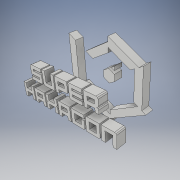
# Autodesk Inventor part: Super-Haxagon
Saved by Autodesk Inventor 2017 (Build 210142000, 142)
## iProperties
Created: 2016-12-10
Part Number: Super-Haxagon
Material: Generic
Document SubType Name: Modeling
Designer: AJ
Density: 1 g/cm^3
Appearance: Default
Author: AJ
Autodesk Inventor part; units mm, degrees
ref_plane "YZ Plane" through (0, 0, 0) normal (1, 0, 0) x (0, 1, 0)
ref_plane "XZ Plane" through (0, 0, 0) normal (0, 1, 0) x (-1, 0, 0)
ref_plane "XY Plane" through (0, 0, 0) normal (0, 0, 1) x (1, 0, 0)
sketch "Shapes" plane through (0, 0, 0) normal (0, 0, 1) x (1, 0, 0)
  circle A0 centre (0, 0) radius 19.05 construction
  line L0 (15.6048, 10.9266) -> (-1.6603, 18.9775)
  line L1 (-1.6603, 18.9775) -> (-17.2652, 8.0509)
  line L2 (-17.2652, 8.0509) -> (-15.6048, -10.9266)
  line L3 (15.6048, 10.9266) -> (17.2652, -8.0509)
  line L4 (17.2652, -8.0509) -> (1.6603, -18.9775)
  line L5 (1.6603, -18.9775) -> (-15.6048, -10.9266)
  line L6 (0, 0) -> (15.6048, 10.9266) construction
  line L7 (0, 0) -> (19.05, 0) construction
  line L8 (6.9723, 14.9521) -> (8.0509, 17.2652) construction
  line L9 (8.0509, 17.2652) -> (10.1978, 21.8692) construction
  line L10 (10.1978, 21.8692) -> (5.5937, 24.0161)
  line L11 (5.5937, 24.0161) -> (14.4916, 31.0773)
  line L12 (14.4916, 31.0773) -> (14.8018, 19.7223)
  line L13 (14.8018, 19.7223) -> (10.1978, 21.8692)
  line L14 (10.1978, 21.8692) -> (14.4916, 31.0773) construction
  line L15 (0, 0) -> (-17.2652, 8.0509) construction
  line L16 (0, 0) -> (-15.6048, -10.9266) construction
  line L17 (0, 0) -> (1.6603, -18.9775) construction
  line L18 (0, 0) -> (17.2652, -8.0509) construction
  line L19 (0, 0) -> (-1.6603, 18.9775) construction
  line L20 (15.6048, 10.9266) -> (46.8145, 32.7799) construction
  line L21 (17.2652, -8.0509) -> (51.7955, -24.1526) construction
  line L22 (1.6603, -18.9775) -> (4.981, -56.9325) construction
  line L23 (-15.6048, -10.9266) -> (-46.8145, -32.7799) construction
  line L24 (-17.2652, 8.0509) -> (-51.7955, 24.1526) construction
  line L25 (-6.0878, 69.5842) -> (57.2178, 40.0643)
  line L26 (78.0242, 54.6332) -> (-8.3016, 94.8875)
  line L27 (67.621, 47.3487) -> (74.8157, -34.8871)
  line L28 (88.4275, 61.9176) -> (97.8359, -45.6216)
  line L29 (86.3258, -40.2544) -> (8.3016, -94.8875)
  line L30 (109.346, -50.9889) -> (10.5153, -120.1909)
  line L31 (9.4085, -107.5392) -> (-88.4275, -61.9176)
  line L32 (11.6222, -132.8426) -> (-109.2339, -76.4864)
  line L33 (-98.8307, -69.202) -> (-109.346, 50.9889)
  line L34 (-132.3663, 61.7234) -> (-119.6372, -83.7708)
  line L35 (-51.7955, 24.1526) -> (-4.981, 56.9325)
  line L36 (-7.1947, 82.2359) -> (-74.8157, 34.8871)
  line L37 (57.2178, 40.0643) -> (78.0242, 54.6332)
  line L38 (67.621, 47.3487) -> (88.4275, 61.9176)
  line L39 (74.8157, -34.8871) -> (97.8359, -45.6216)
  line L40 (86.3258, -40.2544) -> (109.346, -50.9889)
  line L41 (8.3016, -94.8875) -> (10.5153, -120.1909)
  line L42 (9.4085, -107.5392) -> (11.6222, -132.8426)
  line L43 (-119.6372, -83.7708) -> (-98.8307, -69.202)
  line L44 (-109.2339, -76.4864) -> (-88.4275, -61.9176)
  line L45 (-51.7955, 24.1526) -> (-74.8157, 34.8871)
  line L46 (-4.981, 56.9325) -> (-7.1947, 82.2359)
  line L47 (-132.3663, 61.7234) -> (-109.346, 50.9889)
  line L48 (-1.6603, 18.9775) -> (-4.981, 56.9325) construction
  line L49 (-6.0878, 69.5842) -> (-8.3016, 94.8875)
  line L50 (-4.981, 56.9325) -> (-6.0878, 69.5842)
  line L51 (57.2178, 40.0643) -> (67.621, 47.3487)
  line L52 (74.8157, -34.8871) -> (86.3258, -40.2544)
  line L53 (-88.4275, -61.9176) -> (-98.8307, -69.202)
  line L54 (8.3016, -94.8875) -> (9.4085, -107.5392)
  dimension "d0" = 38.1
  dimension "d1" = 35
  dimension "d2" = 5.08
  dimension "d3" = 10.16
  dimension "d4" = 5.08
  dimension "d28" = 38.1
  dimension "d29" = 25.4
  dimension "d30" = 12.7
  dimension "d31" = 12.7
  dimension "d32" = 12.7
  dimension "d33" = 12.7
  dimension "d34" = 12.7
  constraints: 110 end point, 21 collinear, 19 point on line, 16 equal length, 13 parallel, 3 perpendicular, 1 coincident, 1 horizontal, 1 midpoint, 12 other
  measures "d1" angle of L6 L7
  measures "d2" distance of L8.end L9.end
  measures "d3" distance of L9.end L11.end
  measures "d4" distance of L9.end L10.end
  measures "d28" distance of L0.end L48.end
  measures "d29" distance of L35.end L36.start
  measures "d30" distance of L48.end L25.start
  measures "d31" distance of L25.end L27.start
  measures "d32" distance of L27.end L29.start
  measures "d33" distance of L29.end L31.start
  measures "d34" distance of L31.end L33.start
extrude "Hexagon" add sketch "Shapes" along normal blind 25.4
sketch "Lift" plane through (88.4275, 61.9176, 25.4) normal (0.9961947, 0.0871557, 0) x (0, 0, -1)
  line L0 (25.4, 0) -> (0, 0) projected
  line L1 (0, 0) -> (-101.6, 0)
  dimension "d39" = 101.6
  constraints: 2 end point, 1 horizontal
  measures "d39" distance of L0.end L1.end
ref_plane "Offset Face" through (88.4275, 61.9176, 127) normal (0, 0, 1) x (1, 0, 0)
sketch "Words" plane through (88.4275, 61.9176, 127) normal (0, 0, 1) x (1, 0, 0)
  line L0 (-249.7554, -31.6831) -> (43.2861, -6.0452) construction
  line L1 (43.2861, -6.0452) -> (52.3943, -110.1527) construction
  line L2 (52.3943, -110.1527) -> (-240.6472, -135.7905) construction
  line L3 (-240.6472, -135.7905) -> (-249.7554, -31.6831) construction
  line L4 (-240.6472, -135.7905) -> (-209.1715, -133.0367)
  line L5 (52.3943, -110.1527) -> (20.9186, -112.9065)
  line L6 (-220.7937, -0.1942) -> (-208.0646, -145.6884) projected
  line L7 (-204.4757, -65.9671) -> (-205.3069, -56.4668)
  line L8 (-205.3069, -56.4668) -> (-176.829, -53.9753)
  line L9 (-176.829, -53.9753) -> (-177.2426, -49.2483)
  line L10 (-177.2426, -49.2483) -> (-205.7205, -51.7398)
  line L11 (-205.7205, -51.7398) -> (-207.3808, -32.7623)
  spline S0 degree 2 poles (-207.3808, -32.7623) (-207.5531, -30.7927) (-206.3056, -29.306) knots 0 0 0 1 1 1
  spline S1 degree 2 poles (-206.3056, -29.306) (-205.0158, -27.7688) (-203.0462, -27.5965) knots 0 0 0 1 1 1
  line L12 (-203.0462, -27.5965) -> (-169.8413, -24.6915)
  line L13 (-169.8413, -24.6915) -> (-169.0122, -34.1686)
  line L14 (-169.0122, -34.1686) -> (-197.4669, -36.6581)
  line L15 (-197.4669, -36.6581) -> (-197.0513, -41.4083)
  line L16 (-197.0513, -41.4083) -> (-168.5966, -38.9188)
  line L17 (-168.5966, -38.9188) -> (-166.9363, -57.8963)
  spline S2 degree 2 poles (-166.9363, -57.8963) (-166.7599, -59.9123) (-168.0538, -61.403) knots 0 0 0 1 1 1
  spline S3 degree 2 poles (-168.0538, -61.403) (-169.3476, -62.8938) (-171.2709, -63.0621) knots 0 0 0 1 1 1
  line L18 (-171.2709, -63.0621) -> (-204.4757, -65.9671)
  spline S4 degree 2 poles (-157.9009, -61.8924) (-159.9168, -62.0687) (-161.4035, -60.8212) knots 0 0 0 1 1 1
  spline S5 degree 2 poles (-161.4035, -60.8212) (-162.8943, -59.5274) (-163.0666, -57.5578) knots 0 0 0 1 1 1
  line L19 (-163.0666, -57.5578) -> (-165.9717, -24.3529)
  line L20 (-165.9717, -24.3529) -> (-156.4713, -23.5218)
  line L21 (-156.4713, -23.5218) -> (-153.9819, -51.9764)
  line L22 (-153.9819, -51.9764) -> (-135.0044, -50.3161)
  line L23 (-135.0044, -50.3161) -> (-137.4938, -21.8614)
  line L24 (-137.4938, -21.8614) -> (-128.0167, -21.0323)
  line L25 (-128.0167, -21.0323) -> (-124.696, -58.9873)
  line L26 (-124.696, -58.9873) -> (-157.9009, -61.8924)
  line L27 (-120.8264, -58.6488) -> (-124.147, -20.6937)
  line L28 (-124.147, -20.6937) -> (-86.192, -17.3731)
  line L29 (-86.192, -17.3731) -> (-84.1161, -41.1008)
  spline S6 degree 2 poles (-84.1161, -41.1008) (-83.9418, -43.0935) (-85.2356, -44.5843) knots 0 0 0 1 1 1
  spline S7 degree 2 poles (-85.2356, -44.5843) (-86.5295, -46.0751) (-88.4527, -46.2434) knots 0 0 0 1 1 1
  line L30 (-88.4527, -46.2434) -> (-112.1572, -48.3173)
  line L31 (-112.1572, -48.3173) -> (-111.326, -57.8176)
  line L32 (-111.326, -57.8176) -> (-120.8264, -58.6488)
  line L33 (-94.0089, -37.1798) -> (-94.84, -27.6794)
  line L34 (-94.84, -27.6794) -> (-113.8175, -29.3397)
  line L35 (-113.8175, -29.3397) -> (-112.9864, -38.8401)
  line L36 (-112.9864, -38.8401) -> (-94.0089, -37.1798)
  spline S8 degree 2 poles (-74.2515, -54.574) (-76.2675, -54.7504) (-77.7542, -53.5028) knots 0 0 0 1 1 1
  spline S9 degree 2 poles (-77.7542, -53.5028) (-79.245, -52.209) (-79.4173, -50.2394) knots 0 0 0 1 1 1
  line L37 (-79.4173, -50.2394) -> (-82.3224, -17.0346)
  line L38 (-82.3224, -17.0346) -> (-44.3673, -13.7139)
  line L39 (-44.3673, -13.7139) -> (-43.5382, -23.1911)
  line L40 (-43.5382, -23.1911) -> (-71.9929, -25.6806)
  line L41 (-71.9929, -25.6806) -> (-71.5773, -30.4307)
  line L42 (-71.5773, -30.4307) -> (-43.1226, -27.9413)
  line L43 (-43.1226, -27.9413) -> (-42.2914, -37.4416)
  line L44 (-42.2914, -37.4416) -> (-70.7461, -39.9311)
  line L45 (-70.7461, -39.9311) -> (-70.3326, -44.6581)
  line L46 (-70.3326, -44.6581) -> (-41.8779, -42.1686)
  line L47 (-41.8779, -42.1686) -> (-41.0467, -51.6689)
  line L48 (-41.0467, -51.6689) -> (-74.2515, -54.574)
  line L49 (-37.1771, -51.3304) -> (-40.4977, -13.3754)
  line L50 (-40.4977, -13.3754) -> (-7.2928, -10.4703)
  spline S10 degree 2 poles (-7.2928, -10.4703) (-5.3233, -10.298) (-3.8325, -11.5919) knots 0 0 0 1 1 1
  spline S11 degree 2 poles (-3.8325, -11.5919) (-2.2953, -12.8817) (-2.1271, -14.8049) knots 0 0 0 1 1 1
  line L51 (-2.1271, -14.8049) -> (-0.8823, -29.0323)
  spline S12 degree 2 poles (-0.8823, -29.0323) (-0.708, -31.025) (-1.9998, -32.539) knots 0 0 0 1 1 1
  spline S13 degree 2 poles (-1.9998, -32.539) (-3.2937, -34.0297) (-5.2169, -34.198) knots 0 0 0 1 1 1
  spline S14 degree 2 poles (-5.2169, -34.198) (-3.2474, -34.0257) (-1.7566, -35.3195) knots 0 0 0 1 1 1
  spline S15 degree 2 poles (-1.7566, -35.3195) (-0.2215, -36.5862) (-0.0532, -38.5094) knots 0 0 0 1 1 1
  line L52 (-0.0532, -38.5094) -> (0.778, -48.0098)
  line L53 (0.778, -48.0098) -> (-8.6992, -48.8389)
  line L54 (-8.6992, -48.8389) -> (-9.5304, -39.3386)
  line L55 (-9.5304, -39.3386) -> (-28.5079, -40.9989)
  line L56 (-28.5079, -40.9989) -> (-27.6767, -50.4992)
  line L57 (-27.6767, -50.4992) -> (-37.1771, -51.3304)
  line L58 (-10.3595, -29.8614) -> (-11.1907, -20.3611)
  line L59 (-11.1907, -20.3611) -> (-30.1682, -22.0214)
  line L60 (-30.1682, -22.0214) -> (-29.337, -31.5217)
  line L61 (-29.337, -31.5217) -> (-10.3595, -29.8614)
  line L62 (-241.1276, -128.7519) -> (-244.4482, -90.7969)
  line L63 (-244.4482, -90.7969) -> (-234.9479, -89.9657)
  line L64 (-234.9479, -89.9657) -> (-233.7031, -104.1931)
  line L65 (-233.7031, -104.1931) -> (-214.7256, -102.5328)
  line L66 (-214.7256, -102.5328) -> (-215.9703, -88.3054)
  line L67 (-215.9703, -88.3054) -> (-206.4932, -87.4763)
  line L68 (-206.4932, -87.4763) -> (-203.1725, -125.4313)
  line L69 (-203.1725, -125.4313) -> (-212.6497, -126.2604)
  line L70 (-212.6497, -126.2604) -> (-213.8944, -112.0331)
  line L71 (-213.8944, -112.0331) -> (-232.872, -113.6934)
  line L72 (-232.872, -113.6934) -> (-231.6272, -127.9207)
  line L73 (-231.6272, -127.9207) -> (-241.1276, -128.7519)
  line L74 (-199.3029, -125.0927) -> (-202.2079, -91.8879)
  spline S16 degree 2 poles (-202.2079, -91.8879) (-202.3803, -89.9183) (-201.1327, -88.4316) knots 0 0 0 1 1 1
  spline S17 degree 2 poles (-201.1327, -88.4316) (-199.8429, -86.8944) (-197.8734, -86.7221) knots 0 0 0 1 1 1
  line L75 (-197.8734, -86.7221) -> (-164.6685, -83.8171)
  line L76 (-164.6685, -83.8171) -> (-161.3479, -121.7721)
  line L77 (-161.3479, -121.7721) -> (-170.825, -122.6012)
  line L78 (-170.825, -122.6012) -> (-171.6562, -113.1009)
  line L79 (-171.6562, -113.1009) -> (-190.6337, -114.7612)
  line L80 (-190.6337, -114.7612) -> (-189.8026, -124.2616)
  line L81 (-189.8026, -124.2616) -> (-199.3029, -125.0927)
  line L82 (-172.4854, -103.6237) -> (-173.3165, -94.1234)
  line L83 (-173.3165, -94.1234) -> (-192.294, -95.7837)
  line L84 (-192.294, -95.7837) -> (-191.4629, -105.2841)
  line L85 (-191.4629, -105.2841) -> (-172.4854, -103.6237)
  line L86 (-157.4782, -121.4336) -> (-158.723, -107.2062)
  spline S18 degree 2 poles (-158.723, -107.2062) (-158.8953, -105.2366) (-157.6478, -103.7499) knots 0 0 0 1 1 1
  spline S19 degree 2 poles (-157.6478, -103.7499) (-156.358, -102.2128) (-154.3884, -102.0405) knots 0 0 0 1 1 1
  spline S20 degree 2 poles (-154.3884, -102.0405) (-156.4043, -102.2168) (-157.891, -100.9693) knots 0 0 0 1 1 1
  spline S21 degree 2 poles (-157.891, -100.9693) (-159.3818, -99.6755) (-159.5541, -97.7059) knots 0 0 0 1 1 1
  line L87 (-159.5541, -97.7059) -> (-160.7989, -83.4785)
  line L88 (-160.7989, -83.4785) -> (-151.2985, -82.6474)
  line L89 (-151.2985, -82.6474) -> (-150.0538, -96.8747)
  line L90 (-150.0538, -96.8747) -> (-131.0763, -95.2144)
  line L91 (-131.0763, -95.2144) -> (-132.321, -80.987)
  line L92 (-132.321, -80.987) -> (-122.8438, -80.1579)
  line L93 (-122.8438, -80.1579) -> (-121.5991, -94.3852)
  spline S22 degree 2 poles (-121.5991, -94.3852) (-121.4227, -96.4012) (-122.7166, -97.8919) knots 0 0 0 1 1 1
  spline S23 degree 2 poles (-122.7166, -97.8919) (-124.0105, -99.3827) (-125.9337, -99.551) knots 0 0 0 1 1 1
  spline S24 degree 2 poles (-125.9337, -99.551) (-123.9641, -99.3787) (-122.4733, -100.6725) knots 0 0 0 1 1 1
  spline S25 degree 2 poles (-122.4733, -100.6725) (-120.9362, -101.9623) (-120.7679, -103.8856) knots 0 0 0 1 1 1
  line L94 (-120.7679, -103.8856) -> (-119.5232, -118.1129)
  line L95 (-119.5232, -118.1129) -> (-129.0004, -118.9421)
  line L96 (-129.0004, -118.9421) -> (-130.2451, -104.7147)
  line L97 (-130.2451, -104.7147) -> (-149.2226, -106.375)
  line L98 (-149.2226, -106.375) -> (-147.9779, -120.6024)
  line L99 (-147.9779, -120.6024) -> (-157.4782, -121.4336)
  line L100 (-115.6536, -117.7744) -> (-118.5586, -84.5695)
  spline S26 degree 2 poles (-118.5586, -84.5695) (-118.7309, -82.5999) (-117.4834, -81.1132) knots 0 0 0 1 1 1
  spline S27 degree 2 poles (-117.4834, -81.1132) (-116.1936, -79.5761) (-114.224, -79.4038) knots 0 0 0 1 1 1
  line L101 (-114.224, -79.4038) -> (-81.0192, -76.4987)
  line L102 (-81.0192, -76.4987) -> (-77.6985, -114.4537)
  line L103 (-77.6985, -114.4537) -> (-87.1757, -115.2829)
  line L104 (-87.1757, -115.2829) -> (-88.0069, -105.7825)
  line L105 (-88.0069, -105.7825) -> (-106.9844, -107.4429)
  line L106 (-106.9844, -107.4429) -> (-106.1532, -116.9432)
  line L107 (-106.1532, -116.9432) -> (-115.6536, -117.7744)
  line L108 (-88.836, -96.3054) -> (-89.6672, -86.805)
  line L109 (-89.6672, -86.805) -> (-108.6447, -88.4653)
  line L110 (-108.6447, -88.4653) -> (-107.8135, -97.9657)
  line L111 (-107.8135, -97.9657) -> (-88.836, -96.3054)
  line L112 (-73.8289, -114.1152) -> (-77.1495, -76.1602)
  line L113 (-77.1495, -76.1602) -> (-39.1945, -72.8395)
  line L114 (-39.1945, -72.8395) -> (-38.3654, -82.3167)
  line L115 (-38.3654, -82.3167) -> (-66.82, -84.8062)
  line L116 (-66.82, -84.8062) -> (-65.1597, -103.7837)
  line L117 (-65.1597, -103.7837) -> (-46.1822, -102.1234)
  line L118 (-46.1822, -102.1234) -> (-47.4269, -87.896)
  line L119 (-47.4269, -87.896) -> (-37.9498, -87.0669)
  line L120 (-37.9498, -87.0669) -> (-36.2895, -106.0444)
  spline S28 degree 2 poles (-36.2895, -106.0444) (-36.1131, -108.0603) (-37.4069, -109.5511) knots 0 0 0 1 1 1
  spline S29 degree 2 poles (-37.4069, -109.5511) (-38.7008, -111.0419) (-40.624, -111.2101) knots 0 0 0 1 1 1
  line L121 (-40.624, -111.2101) -> (-73.8289, -114.1152)
  line L122 (-32.0042, -110.456) -> (-34.9093, -77.2511)
  spline S30 degree 2 poles (-34.9093, -77.2511) (-35.0816, -75.2816) (-33.8341, -73.7948) knots 0 0 0 1 1 1
  spline S31 degree 2 poles (-33.8341, -73.7948) (-32.5443, -72.2577) (-30.5747, -72.0854) knots 0 0 0 1 1 1
  line L123 (-30.5747, -72.0854) -> (2.6302, -69.1803)
  line L124 (2.6302, -69.1803) -> (5.5352, -102.3852)
  spline S32 degree 2 poles (5.5352, -102.3852) (5.7116, -104.4011) (4.4177, -105.8919) knots 0 0 0 1 1 1
  spline S33 degree 2 poles (4.4177, -105.8919) (3.1239, -107.3827) (1.2006, -107.5509) knots 0 0 0 1 1 1
  line L125 (1.2006, -107.5509) -> (-32.0042, -110.456)
  line L126 (-4.3575, -98.4642) -> (-6.0179, -79.4867)
  line L127 (-6.0179, -79.4867) -> (-24.9954, -81.147)
  line L128 (-24.9954, -81.147) -> (-23.3351, -100.1245)
  line L129 (-23.3351, -100.1245) -> (-4.3575, -98.4642)
  line L130 (9.8204, -106.7968) -> (6.4998, -68.8418)
  line L131 (6.4998, -68.8418) -> (39.7047, -65.9367)
  spline S34 degree 2 poles (39.7047, -65.9367) (41.6742, -65.7644) (43.165, -67.0583) knots 0 0 0 1 1 1
  spline S35 degree 2 poles (43.165, -67.0583) (44.7022, -68.3481) (44.8704, -70.2713) knots 0 0 0 1 1 1
  line L132 (44.8704, -70.2713) -> (47.7755, -103.4762)
  line L133 (47.7755, -103.4762) -> (38.2983, -104.3053)
  line L134 (38.2983, -104.3053) -> (35.8068, -75.8275)
  line L135 (35.8068, -75.8275) -> (16.8293, -77.4878)
  line L136 (16.8293, -77.4878) -> (19.3208, -105.9656)
  line L137 (19.3208, -105.9656) -> (9.8204, -106.7968)
  point P0 (20.9186, -112.9065)
  constraints: 4 end point, 3 point on line, 2 coincident, 1 collinear, 2 other
extrude "Text" add sketch "Words" along normal blind 25.4
body "Solid2"
